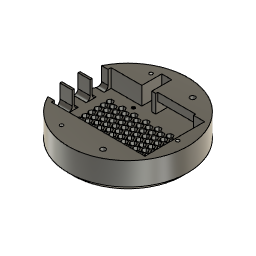
Lumo Base (Autodesk Fusion 360 design; units mm, degrees)
Autodesk Fusion 360 part; units mm, degrees
(part 1 of 2)
sketch "Pi Bounds" plane through (0, 0, 0) normal (0, 0, 1) x (1, 0, 0)
  circle A0 centre (0, 0) radius 60
  line L0 (-47, -30) -> (47, -30)
  line L1 (47, -30) -> (47, 30)
  line L2 (47, 30) -> (-47, 30)
  line L3 (-47, 30) -> (-47, -30)
  line L4 (-47, -30) -> (47, 30) construction
  line L5 (47, -30) -> (-47, 30) construction
  dimension "d1" = 60
  dimension "d2" = 94
  dimension "d3" = 120
  constraint coincident A0.centre origin
  constraint horizontal L0
  constraint perpendicular L0 L1
  constraint parallel L0 L2
  constraint parallel L1 L3
  constraint coincident L4 A0.centre
  constraint coincident L5 A0.centre
  measures "d1" distance of L0.end L1.end
  measures "d2" distance of L1.end L2.end
  measures "d3" diameter of A0
extrude "Extrude1" add sketch "Pi Bounds" along normal blind 28
extrude "Extrude2" add sketch "Pi Bounds" along normal blind 10 contours L0 L1 L2 L3
chamfer "Chamfer1" distance 5 angle 45 1 edges at (-55.9396, -21.6969, 0)
sketch "Screw Holes" plane through (0, 0, 10) normal (0, 0, 1) x (-1, 0, 0)
  line L0 (47, -30) -> (47, 30)
  line L1 (47, 30) -> (-47, 30)
  line L2 (-47, -30) -> (47, -30)
  line L3 (-47, -30) -> (-47, 30)
  point P0 (-39, 24.5)
  point P1 (-39, -24.5)
  point P2 (19, -24.5)
  point P3 (19, 24.5)
  dimension "d35" = 58
  dimension "d36" = 49
  dimension "d144" = 24.5
  dimension "d145" = 39
  dimension "d146" = 8
  constraint vertical P0 P1
  constraint horizontal P0 P3
  constraint vertical P2 P3
  constraint horizontal P1 P2
  measures "d35" distance of P0 P3
  measures "d36" distance of P0 P1
  measures "d144" vertical distance of origin P0
  measures "d145" horizontal distance of origin P0
  measures "d146" distance of P0 L3
hole "Hole3" at (-19, -24.5, 10) at (-19, 24.5, 10) at (39, 24.5, 10) at (39, -24.5, 10) direction (0, 0, -1) diameter 2.529 depth 6 tip angle 180
thread "Thread1" "ISO Metric profile 3.0 M3x0.5 6H" major diameter 3.086 minor diameter 2.529 pitch 0.5 angle 60 modelled right hand crest width 0.1368 on face at (-18.937, -25.7629, 8) crest through (-17.7355, -24.5, 9.875) on face at (-18.937, 23.2371, 8) crest through (-17.7355, 24.5, 9.875) on face at (38.3406, 23.421, 8) crest through (40.2645, 24.5, 9.875) on face at (38.2365, -25.508, 8) crest through (40.2645, -24.5, 9.875)
sketch "Access Holes (Side)" plane through (0, 30, 0) normal (0, -1, 0) x (1, 0, 0)
  line L0 (-47, 10) -> (47, 10)
  line L1 (47, 10) -> (47, 28)
  line L2 (47, 28) -> (-47, 28)
  line L3 (-47, 28) -> (-47, 10)
  line L4 (35.8, 20) -> (25.8, 20)
  line L5 (25.8, 20) -> (25.8, 10)
  line L6 (25.8, 10) -> (35.8, 10)
  line L7 (35.8, 10) -> (35.8, 20)
  line L8 (35.8, 20) -> (25.8, 10) construction
  line L9 (25.8, 20) -> (35.8, 10) construction
  line L10 (21, 10) -> (11, 10)
  line L11 (11, 10) -> (11, 20)
  line L12 (11, 20) -> (21, 20)
  line L13 (21, 20) -> (21, 10)
  line L14 (21, 10) -> (11, 20) construction
  line L15 (11, 10) -> (21, 20) construction
  line L16 (7.869, 20) -> (-2.131, 20)
  line L17 (-2.131, 20) -> (-2.131, 10)
  line L18 (-2.131, 10) -> (7.869, 10)
  line L19 (7.869, 10) -> (7.869, 20)
  line L20 (7.869, 20) -> (-2.131, 10) construction
  line L21 (-2.131, 20) -> (7.869, 10) construction
  line L22 (35.8, 10) -> (-2.131, 10)
  line L23 (-2.131, 10) -> (-2.131, 20)
  line L24 (-2.131, 20) -> (35.8, 20)
  line L25 (35.8, 20) -> (35.8, 10)
  point P0 (30.8, 15)
  point P1 (30.8, 15)
  point P2 (16, 15)
  point P3 (16, 15)
  point P4 (2.5, 15)
  point P5 (2.869, 15)
  dimension "d61" = 16.2
  dimension "d62" = 10
  dimension "d63" = 10
  dimension "d64" = 5
  dimension "d66" = 14.8
  dimension "d67" = 10
  dimension "d68" = 10
  dimension "d69" = 13.5
  dimension "d70" = 10
  dimension "d71" = 10
  constraint horizontal L4
  constraint perpendicular L4 L5
  constraint parallel L4 L6
  constraint parallel L5 L7
  constraint coincident L8 P1
  constraint coincident L9 P1
  constraint coincident P1 P0
  constraint horizontal P1 P3
  constraint horizontal L10
  constraint perpendicular L10 L11
  constraint parallel L10 L12
  constraint parallel L11 L13
  constraint coincident L14 P3
  constraint coincident L15 P3
  constraint coincident P3 P2
  constraint horizontal P3 P4
  constraint horizontal L16
  constraint perpendicular L16 L17
  constraint parallel L16 L18
  constraint parallel L17 L19
  constraint coincident L20 P5
  constraint coincident L21 P5
  constraint horizontal P3 P5
  constraint horizontal L22
  constraint vertical L23
  constraint horizontal L24
  constraint vertical L25
  measures "d61" distance of L1 P1
  measures "d62" distance of L5.end L6.end
  measures "d63" distance of L4.end L5.end
  measures "d64" distance of L0 P1
  measures "d66" distance of P1 P3
  measures "d67" distance of L11.end L12.end
  measures "d68" distance of L10.end L11.end
  measures "d69" distance of P3 P4
  measures "d70" distance of L17.end L18.end
  measures "d71" distance of L16.end L17.end
extrude "Extrude4" cut sketch "Access Holes (Side)" against normal through all contours L0 L16 L17 L18 L19 L22 L23 L24 | L0 L11 L19 L22 L24 | L0 L10 L11 L12 L13 L22 L24 | L0 L5 L13 L22 L24 | L0 L4 L5 L6 L7 L22 L24 L25
sketch "Connectors/Feet" plane through (0, 0, 0) normal (0, 0, -1) x (1, 0, 0)
  circle A0 centre (0, 0) radius 55
  circle A1 centre (0, 0) radius 50
  line L0 (40, -40) -> (-40, -40)
  line L1 (-40, -40) -> (-40, 40)
  line L2 (-40, 40) -> (40, 40)
  line L3 (40, 40) -> (40, -40)
  line L4 (40, -40) -> (-40, 40) construction
  line L5 (-40, -40) -> (40, 40) construction
  point P0 (50, 0)
  point P1 (-21.7945, 45)
  point P2 (-21.7945, -45)
  dimension "d138" = 100
  dimension "d141" = 45
  dimension "d142" = 80
  dimension "d143" = 80
  constraint coincident A0.centre A1.centre
  constraint coincident A1 P0
  constraint coincident A1 P1
  constraint vertical P1 P2
  constraint coincident A1 P2
  constraint horizontal L0
  constraint perpendicular L0 L1
  constraint parallel L0 L2
  constraint parallel L1 L3
  constraint coincident L4 A0.centre
  constraint coincident L5 A0.centre
  measures "d138" diameter of A1
  measures "d141" vertical distance of A0.centre P1
  measures "d142" distance of L1.end L2.end
  measures "d143" distance of L0.end L1.end
hole "Hole4" at (-21.7945, 45, 0) at (-21.7945, -45, 0) at (50, 0, 0) direction (0, 0, 1) diameter 3.332 end through all counterbore diameter 8 counterbore depth 2
thread "Thread2" "ISO Metric profile 4.0 M4x0.7 6H" major diameter 4.1095 minor diameter 3.332 pitch 0.7 angle 60 resizes the face on face at (-21.6286, -43.3423, 10.6667) on face at (50.1659, 1.6577, 10.6667) on face at (-21.6286, 46.6577, 10.6667)
sketch "Hexagon Air Holes" plane through (0, 0, 10) normal (0, 0, 1) x (-1, 0, 0)
  arc A0 (18.0419, 23.6748) -> (19.9581, 23.6748) centre (19, 24.5) ccw
  spline S0 degree 3 poles (18.0419, 23.6748) (17.9198, 23.7888) (17.8216, 23.926) (17.6793, 24.236) (17.6389, 24.407) (17.6243, 24.7618) (17.6529, 24.9423) (17.7788, 25.2891) (17.8774, 25.4512) (18.0844, 25.6792) (18.1756, 25.7577) (18.3768, 25.8929) (18.4864, 25.9486) (18.6015, 25.9906) knots 0 0 0 0 0.050111 0.050111 0.102261 0.102261 0.15645 0.15645 0.212677 0.212677 0.24852 0.24852 0.285143 0.285143 0.285143 0.285143
  arc A1 (-39.9581, 23.6748) -> (-38.0419, 23.6748) centre (-39, 24.5) ccw
  arc A2 (18.0419, -25.3252) -> (19.9581, -25.3252) centre (19, -24.5) ccw
  arc A3 (-39.9581, -25.3252) -> (-38.0419, -25.3252) centre (-39, -24.5) ccw
  line L0 (47, -30) -> (47, 30)
  line L1 (47, 30) -> (-47, 30)
  line L2 (-47, 30) -> (-47, -30)
  line L3 (-47, -30) -> (-35.8, -30)
  line L4 (33, -18.088) -> (34.5, -20.6861)
  line L5 (34.5, -20.6861) -> (37.5, -20.6861)
  line L6 (37.5, -20.6861) -> (39, -18.088)
  line L7 (39, -18.088) -> (37.5, -15.4899)
  line L8 (37.5, -15.4899) -> (34.5, -15.4899)
  line L9 (34.5, -15.4899) -> (33, -18.088)
  line L10 (34.5, -14.4901) -> (37.5, -14.4901)
  line L11 (37.5, -14.4901) -> (39, -11.892)
  line L12 (39, -11.892) -> (37.5, -9.2939)
  line L13 (37.5, -9.2939) -> (34.5, -9.2939)
  line L14 (34.5, -9.2939) -> (33, -11.892)
  line L15 (33, -11.892) -> (34.5, -14.4901)
  line L16 (34.5, -8.2941) -> (37.5, -8.2941)
  line L17 (37.5, -8.2941) -> (39, -5.696)
  line L18 (39, -5.696) -> (37.5, -3.0979)
  line L19 (37.5, -3.0979) -> (34.5, -3.0979)
  line L20 (34.5, -3.0979) -> (33, -5.696)
  line L21 (33, -5.696) -> (34.5, -8.2941)
  line L22 (34.5, -2.0981) -> (37.5, -2.0981)
  line L23 (37.5, -2.0981) -> (39, 0.5)
  line L24 (39, 0.5) -> (37.5, 3.0981)
  line L25 (37.5, 3.0981) -> (34.5, 3.0981)
  line L26 (34.5, 3.0981) -> (33, 0.5)
  line L27 (33, 0.5) -> (34.5, -2.0981)
  line L28 (34.5, 4.0979) -> (37.5, 4.0979)
  line L29 (37.5, 4.0979) -> (39, 6.696)
  line L30 (39, 6.696) -> (37.5, 9.2941)
  line L31 (37.5, 9.2941) -> (34.5, 9.2941)
  line L32 (34.5, 9.2941) -> (33, 6.696)
  line L33 (33, 6.696) -> (34.5, 4.0979)
  line L34 (34.5, 10.2939) -> (37.5, 10.2939)
  line L35 (37.5, 10.2939) -> (39, 12.892)
  line L36 (39, 12.892) -> (37.5, 15.4901)
  line L37 (37.5, 15.4901) -> (34.5, 15.4901)
  line L38 (34.5, 15.4901) -> (33, 12.892)
  line L39 (33, 12.892) -> (34.5, 10.2939)
  line L40 (34.5, 16.4899) -> (37.5, 16.4899)
  line L41 (37.5, 16.4899) -> (39, 19.088)
  line L42 (39, 19.088) -> (37.5, 21.6861)
  line L43 (37.5, 21.6861) -> (34.5, 21.6861)
  line L44 (34.5, 21.6861) -> (33, 19.088)
  line L45 (33, 19.088) -> (34.5, 16.4899)
  line L46 (21, -18.088) -> (22.5, -20.6861)
  line L47 (22.5, -20.6861) -> (25.5, -20.6861)
  line L48 (25.5, -20.6861) -> (27, -18.088)
  line L49 (27, -18.088) -> (25.5, -15.4899)
  line L50 (22.5, -15.4899) -> (21, -18.088)
  line L51 (25.5, -15.4899) -> (22.5, -15.4899)
  line L52 (25.5, -9.2939) -> (22.5, -9.2939)
  line L53 (22.5, -9.2939) -> (21, -11.892)
  line L54 (21, -11.892) -> (22.5, -14.4901)
  line L55 (22.5, -14.4901) -> (25.5, -14.4901)
  line L56 (27, -11.892) -> (25.5, -9.2939)
  line L57 (25.5, -14.4901) -> (27, -11.892)
  line L58 (25.5, -3.0979) -> (22.5, -3.0979)
  line L59 (22.5, -3.0979) -> (21, -5.696)
  line L60 (21, -5.696) -> (22.5, -8.2941)
  line L61 (22.5, -8.2941) -> (25.5, -8.2941)
  line L62 (27, -5.696) -> (25.5, -3.0979)
  line L63 (25.5, -8.2941) -> (27, -5.696)
  line L64 (25.5, 3.0981) -> (22.5, 3.0981)
  line L65 (22.5, 3.0981) -> (21, 0.5)
  line L66 (21, 0.5) -> (22.5, -2.0981)
  line L67 (22.5, -2.0981) -> (25.5, -2.0981)
  line L68 (27, 0.5) -> (25.5, 3.0981)
  line L69 (25.5, -2.0981) -> (27, 0.5)
  line L70 (27, 6.696) -> (25.5, 9.2941)
  line L71 (25.5, 9.2941) -> (22.5, 9.2941)
  line L72 (22.5, 9.2941) -> (21, 6.696)
  line L73 (21, 6.696) -> (22.5, 4.0979)
  line L74 (25.5, 4.0979) -> (27, 6.696)
  line L75 (22.5, 4.0979) -> (25.5, 4.0979)
  line L76 (27, 12.892) -> (25.5, 15.4901)
  line L77 (25.5, 15.4901) -> (22.5, 15.4901)
  line L78 (22.5, 15.4901) -> (21, 12.892)
  line L79 (21, 12.892) -> (22.5, 10.2939)
  line L80 (25.5, 10.2939) -> (27, 12.892)
  line L81 (22.5, 10.2939) -> (25.5, 10.2939)
  line L82 (27, 19.088) -> (25.5, 21.6861)
  line L83 (25.5, 21.6861) -> (22.5, 21.6861)
  line L84 (22.5, 21.6861) -> (21, 19.088)
  line L85 (21, 19.088) -> (22.5, 16.4899)
  line L86 (25.5, 16.4899) -> (27, 19.088)
  line L87 (22.5, 16.4899) -> (25.5, 16.4899)
  line L88 (9, -18.088) -> (10.5, -20.6861)
  line L89 (10.5, -20.6861) -> (13.5, -20.6861)
  line L90 (13.5, -20.6861) -> (15, -18.088)
  line L91 (15, -18.088) -> (13.5, -15.4899)
  line L92 (10.5, -15.4899) -> (9, -18.088)
  line L93 (13.5, -15.4899) -> (10.5, -15.4899)
  line L94 (13.5, -9.2939) -> (10.5, -9.2939)
  line L95 (10.5, -9.2939) -> (9, -11.892)
  line L96 (9, -11.892) -> (10.5, -14.4901)
  line L97 (10.5, -14.4901) -> (13.5, -14.4901)
  line L98 (15, -11.892) -> (13.5, -9.2939)
  line L99 (13.5, -14.4901) -> (15, -11.892)
  line L100 (13.5, -3.0979) -> (10.5, -3.0979)
  line L101 (10.5, -3.0979) -> (9, -5.696)
  line L102 (9, -5.696) -> (10.5, -8.2941)
  line L103 (10.5, -8.2941) -> (13.5, -8.2941)
  line L104 (15, -5.696) -> (13.5, -3.0979)
  line L105 (13.5, -8.2941) -> (15, -5.696)
  line L106 (13.5, 3.0981) -> (10.5, 3.0981)
  line L107 (10.5, 3.0981) -> (9, 0.5)
  line L108 (9, 0.5) -> (10.5, -2.0981)
  line L109 (10.5, -2.0981) -> (13.5, -2.0981)
  line L110 (15, 0.5) -> (13.5, 3.0981)
  line L111 (13.5, -2.0981) -> (15, 0.5)
  line L112 (15, 6.696) -> (13.5, 9.2941)
  line L113 (13.5, 9.2941) -> (10.5, 9.2941)
  line L114 (10.5, 9.2941) -> (9, 6.696)
  line L115 (9, 6.696) -> (10.5, 4.0979)
  line L116 (13.5, 4.0979) -> (15, 6.696)
  line L117 (10.5, 4.0979) -> (13.5, 4.0979)
  line L118 (15, 12.892) -> (13.5, 15.4901)
  line L119 (13.5, 15.4901) -> (10.5, 15.4901)
  line L120 (10.5, 15.4901) -> (9, 12.892)
  line L121 (9, 12.892) -> (10.5, 10.2939)
  line L122 (13.5, 10.2939) -> (15, 12.892)
  line L123 (10.5, 10.2939) -> (13.5, 10.2939)
  line L124 (15, 19.088) -> (13.5, 21.6861)
  line L125 (13.5, 21.6861) -> (10.5, 21.6861)
  line L126 (10.5, 21.6861) -> (9, 19.088)
  line L127 (9, 19.088) -> (10.5, 16.4899)
  line L128 (13.5, 16.4899) -> (15, 19.088)
  line L129 (10.5, 16.4899) -> (13.5, 16.4899)
  line L130 (-3, -18.088) -> (-1.5, -20.6861)
  line L131 (-1.5, -20.6861) -> (1.5, -20.6861)
  line L132 (1.5, -20.6861) -> (3, -18.088)
  line L133 (3, -18.088) -> (1.5, -15.4899)
  line L134 (-1.5, -15.4899) -> (-3, -18.088)
  line L135 (1.5, -15.4899) -> (-1.5, -15.4899)
  line L136 (1.5, -9.2939) -> (-1.5, -9.2939)
  line L137 (-1.5, -9.2939) -> (-3, -11.892)
  line L138 (-3, -11.892) -> (-1.5, -14.4901)
  line L139 (-1.5, -14.4901) -> (1.5, -14.4901)
  line L140 (3, -11.892) -> (1.5, -9.2939)
  line L141 (1.5, -14.4901) -> (3, -11.892)
  line L142 (1.5, -3.0979) -> (-1.5, -3.0979)
  line L143 (-1.5, -3.0979) -> (-3, -5.696)
  line L144 (-3, -5.696) -> (-1.5, -8.2941)
  line L145 (-1.5, -8.2941) -> (1.5, -8.2941)
  line L146 (3, -5.696) -> (1.5, -3.0979)
  line L147 (1.5, -8.2941) -> (3, -5.696)
  line L148 (1.5, 3.0981) -> (-1.5, 3.0981)
  line L149 (-1.5, 3.0981) -> (-3, 0.5)
  line L150 (-3, 0.5) -> (-1.5, -2.0981)
  line L151 (-1.5, -2.0981) -> (1.5, -2.0981)
  line L152 (3, 0.5) -> (1.5, 3.0981)
  line L153 (1.5, -2.0981) -> (3, 0.5)
  line L154 (3, 6.696) -> (1.5, 9.2941)
  line L155 (1.5, 9.2941) -> (-1.5, 9.2941)
  line L156 (-1.5, 9.2941) -> (-3, 6.696)
  line L157 (-3, 6.696) -> (-1.5, 4.0979)
  line L158 (1.5, 4.0979) -> (3, 6.696)
  line L159 (-1.5, 4.0979) -> (1.5, 4.0979)
  line L160 (3, 12.892) -> (1.5, 15.4901)
  line L161 (1.5, 15.4901) -> (-1.5, 15.4901)
  line L162 (-1.5, 15.4901) -> (-3, 12.892)
  line L163 (-3, 12.892) -> (-1.5, 10.2939)
  line L164 (1.5, 10.2939) -> (3, 12.892)
  line L165 (-1.5, 10.2939) -> (1.5, 10.2939)
  line L166 (3, 19.088) -> (1.5, 21.6861)
  line L167 (1.5, 21.6861) -> (-1.5, 21.6861)
  line L168 (-1.5, 21.6861) -> (-3, 19.088)
  line L169 (-3, 19.088) -> (-1.5, 16.4899)
  line L170 (1.5, 16.4899) -> (3, 19.088)
  line L171 (-1.5, 16.4899) -> (1.5, 16.4899)
  line L172 (-15, -18.088) -> (-13.5, -20.6861)
  line L173 (-13.5, -20.6861) -> (-10.5, -20.6861)
  line L174 (-10.5, -20.6861) -> (-9, -18.088)
  line L175 (-9, -18.088) -> (-10.5, -15.4899)
  line L176 (-13.5, -15.4899) -> (-15, -18.088)
  line L177 (-10.5, -15.4899) -> (-13.5, -15.4899)
  line L178 (-10.5, -9.2939) -> (-13.5, -9.2939)
  line L179 (-13.5, -9.2939) -> (-15, -11.892)
  line L180 (-15, -11.892) -> (-13.5, -14.4901)
  line L181 (-13.5, -14.4901) -> (-10.5, -14.4901)
  line L182 (-9, -11.892) -> (-10.5, -9.2939)
  line L183 (-10.5, -14.4901) -> (-9, -11.892)
  line L184 (-10.5, -3.0979) -> (-13.5, -3.0979)
  line L185 (-13.5, -3.0979) -> (-15, -5.696)
  line L186 (-15, -5.696) -> (-13.5, -8.2941)
  line L187 (-13.5, -8.2941) -> (-10.5, -8.2941)
  line L188 (-9, -5.696) -> (-10.5, -3.0979)
  line L189 (-10.5, -8.2941) -> (-9, -5.696)
  line L190 (-10.5, 3.0981) -> (-13.5, 3.0981)
  line L191 (-13.5, 3.0981) -> (-15, 0.5)
  line L192 (-15, 0.5) -> (-13.5, -2.0981)
  line L193 (-13.5, -2.0981) -> (-10.5, -2.0981)
  line L194 (-9, 0.5) -> (-10.5, 3.0981)
  line L195 (-10.5, -2.0981) -> (-9, 0.5)
  line L196 (-9, 6.696) -> (-10.5, 9.2941)
  line L197 (-10.5, 9.2941) -> (-13.5, 9.2941)
  line L198 (-13.5, 9.2941) -> (-15, 6.696)
  line L199 (-15, 6.696) -> (-13.5, 4.0979)
  line L200 (-10.5, 4.0979) -> (-9, 6.696)
  line L201 (-13.5, 4.0979) -> (-10.5, 4.0979)
  line L202 (-9, 12.892) -> (-10.5, 15.4901)
  line L203 (-10.5, 15.4901) -> (-13.5, 15.4901)
  line L204 (-13.5, 15.4901) -> (-15, 12.892)
  line L205 (-15, 12.892) -> (-13.5, 10.2939)
  line L206 (-10.5, 10.2939) -> (-9, 12.892)
  line L207 (-13.5, 10.2939) -> (-10.5, 10.2939)
  line L208 (-9, 19.088) -> (-10.5, 21.6861)
  line L209 (-10.5, 21.6861) -> (-13.5, 21.6861)
  line L210 (-13.5, 21.6861) -> (-15, 19.088)
  line L211 (-15, 19.088) -> (-13.5, 16.4899)
  line L212 (-10.5, 16.4899) -> (-9, 19.088)
  line L213 (-13.5, 16.4899) -> (-10.5, 16.4899)
  line L214 (-27, -18.088) -> (-25.5, -20.6861)
  line L215 (-25.5, -20.6861) -> (-22.5, -20.6861)
  line L216 (-22.5, -20.6861) -> (-21, -18.088)
  line L217 (-21, -18.088) -> (-22.5, -15.4899)
  line L218 (-25.5, -15.4899) -> (-27, -18.088)
  line L219 (-22.5, -15.4899) -> (-25.5, -15.4899)
  line L220 (-22.5, -9.2939) -> (-25.5, -9.2939)
  line L221 (-25.5, -9.2939) -> (-27, -11.892)
  line L222 (-27, -11.892) -> (-25.5, -14.4901)
  line L223 (-25.5, -14.4901) -> (-22.5, -14.4901)
  line L224 (-21, -11.892) -> (-22.5, -9.2939)
  line L225 (-22.5, -14.4901) -> (-21, -11.892)
  line L226 (-22.5, -3.0979) -> (-25.5, -3.0979)
  line L227 (-25.5, -3.0979) -> (-27, -5.696)
  line L228 (-27, -5.696) -> (-25.5, -8.2941)
  line L229 (-25.5, -8.2941) -> (-22.5, -8.2941)
  line L230 (-21, -5.696) -> (-22.5, -3.0979)
  line L231 (-22.5, -8.2941) -> (-21, -5.696)
  line L232 (-22.5, 3.0981) -> (-25.5, 3.0981)
  line L233 (-25.5, 3.0981) -> (-27, 0.5)
  line L234 (-27, 0.5) -> (-25.5, -2.0981)
  line L235 (-25.5, -2.0981) -> (-22.5, -2.0981)
  line L236 (-21, 0.5) -> (-22.5, 3.0981)
  line L237 (-22.5, -2.0981) -> (-21, 0.5)
  line L238 (-21, 6.696) -> (-22.5, 9.2941)
  line L239 (-22.5, 9.2941) -> (-25.5, 9.2941)
  line L240 (-25.5, 9.2941) -> (-27, 6.696)
  line L241 (-27, 6.696) -> (-25.5, 4.0979)
  line L242 (-22.5, 4.0979) -> (-21, 6.696)
  line L243 (-25.5, 4.0979) -> (-22.5, 4.0979)
  line L244 (-21, 12.892) -> (-22.5, 15.4901)
  line L245 (-22.5, 15.4901) -> (-25.5, 15.4901)
  line L246 (-25.5, 15.4901) -> (-27, 12.892)
  line L247 (-27, 12.892) -> (-25.5, 10.2939)
  line L248 (-22.5, 10.2939) -> (-21, 12.892)
  line L249 (-25.5, 10.2939) -> (-22.5, 10.2939)
  line L250 (-21, 19.088) -> (-22.5, 21.6861)
  line L251 (-22.5, 21.6861) -> (-25.5, 21.6861)
  line L252 (-25.5, 21.6861) -> (-27, 19.088)
  line L253 (-27, 19.088) -> (-25.5, 16.4899)
  line L254 (-22.5, 16.4899) -> (-21, 19.088)
  line L255 (-25.5, 16.4899) -> (-22.5, 16.4899)
  line L256 (31.5, -17.5881) -> (33, -14.99)
  line L257 (33, -14.99) -> (31.5, -12.3919)
  line L258 (31.5, -12.3919) -> (28.5, -12.3919)
  line L259 (28.5, -12.3919) -> (27, -14.99)
  line L260 (27, -14.99) -> (28.5, -17.5881)
  line L261 (28.5, -17.5881) -> (31.5, -17.5881)
  line L262 (-47, -30) -> (47, -30)
  line L263 (30, -14.99) -> (36, -18.088)
  line L264 (25.5, -20.6861) -> (22.5, -15.4899)
  line L265 (30, -14.99) -> (24, -18.088)
  line L266 (37.5, -14.4901) -> (34.5, -9.2939)
  line L267 (36, -11.892) -> (30, -14.99)
  line L268 (15, -14.99) -> (16.5, -17.5881)
  line L269 (16.5, -17.5881) -> (19.5, -17.5881)
  line L270 (19.5, -17.5881) -> (21, -14.99)
  line L271 (21, -14.99) -> (19.5, -12.3919)
  line L272 (16.5, -12.3919) -> (15, -14.99)
  line L273 (19.5, -12.3919) -> (16.5, -12.3919)
  line L274 (3, -14.99) -> (4.5, -17.5881)
  line L275 (4.5, -17.5881) -> (7.5, -17.5881)
  line L276 (7.5, -17.5881) -> (9, -14.99)
  line L277 (9, -14.99) -> (7.5, -12.3919)
  line L278 (4.5, -12.3919) -> (3, -14.99)
  line L279 (7.5, -12.3919) -> (4.5, -12.3919)
  line L280 (-9, -14.99) -> (-7.5, -17.5881)
  line L281 (-7.5, -17.5881) -> (-4.5, -17.5881)
  line L282 (-4.5, -17.5881) -> (-3, -14.99)
  line L283 (-3, -14.99) -> (-4.5, -12.3919)
  line L284 (-7.5, -12.3919) -> (-9, -14.99)
  line L285 (-4.5, -12.3919) -> (-7.5, -12.3919)
  line L286 (-21, -14.99) -> (-19.5, -17.5881)
  line L287 (-19.5, -17.5881) -> (-16.5, -17.5881)
  line L288 (-16.5, -17.5881) -> (-15, -14.99)
  line L289 (-15, -14.99) -> (-16.5, -12.3919)
  line L290 (-19.5, -12.3919) -> (-21, -14.99)
  line L291 (-16.5, -12.3919) -> (-19.5, -12.3919)
  line L292 (-33, -14.99) -> (-31.5, -17.5881)
  line L293 (-31.5, -17.5881) -> (-28.5, -17.5881)
  line L294 (-28.5, -17.5881) -> (-27, -14.99)
  line L295 (-27, -14.99) -> (-28.5, -12.3919)
  line L296 (-31.5, -12.3919) -> (-33, -14.99)
  line L297 (-28.5, -12.3919) -> (-31.5, -12.3919)
  line L298 (27, -8.821) -> (28.5, -11.4191)
  line L299 (28.5, -11.4191) -> (31.5, -11.4191)
  line L300 (31.5, -11.4191) -> (33, -8.821)
  line L301 (33, -8.821) -> (31.5, -6.2229)
  line L302 (28.5, -6.2229) -> (27, -8.821)
  line L303 (31.5, -6.2229) -> (28.5, -6.2229)
  line L304 (15, -8.821) -> (16.5, -11.4191)
  line L305 (16.5, -11.4191) -> (19.5, -11.4191)
  line L306 (19.5, -11.4191) -> (21, -8.821)
  line L307 (21, -8.821) -> (19.5, -6.2229)
  line L308 (16.5, -6.2229) -> (15, -8.821)
  line L309 (19.5, -6.2229) -> (16.5, -6.2229)
  line L310 (3, -8.821) -> (4.5, -11.4191)
  line L311 (4.5, -11.4191) -> (7.5, -11.4191)
  line L312 (7.5, -11.4191) -> (9, -8.821)
  line L313 (9, -8.821) -> (7.5, -6.2229)
  line L314 (4.5, -6.2229) -> (3, -8.821)
  line L315 (7.5, -6.2229) -> (4.5, -6.2229)
  line L316 (-9, -8.821) -> (-7.5, -11.4191)
  line L317 (-7.5, -11.4191) -> (-4.5, -11.4191)
  line L318 (-4.5, -11.4191) -> (-3, -8.821)
  line L319 (-3, -8.821) -> (-4.5, -6.2229)
  line L320 (-7.5, -6.2229) -> (-9, -8.821)
  line L321 (-4.5, -6.2229) -> (-7.5, -6.2229)
  line L322 (-21, -8.821) -> (-19.5, -11.4191)
  line L323 (-19.5, -11.4191) -> (-16.5, -11.4191)
  line L324 (-16.5, -11.4191) -> (-15, -8.821)
  line L325 (-15, -8.821) -> (-16.5, -6.2229)
  line L326 (-19.5, -6.2229) -> (-21, -8.821)
  line L327 (-16.5, -6.2229) -> (-19.5, -6.2229)
  line L328 (-33, -8.821) -> (-31.5, -11.4191)
  line L329 (-31.5, -11.4191) -> (-28.5, -11.4191)
  line L330 (-28.5, -11.4191) -> (-27, -8.821)
  line L331 (-27, -8.821) -> (-28.5, -6.2229)
  line L332 (-31.5, -6.2229) -> (-33, -8.821)
  line L333 (-28.5, -6.2229) -> (-31.5, -6.2229)
  line L334 (27, -2.652) -> (28.5, -5.2501)
  line L335 (28.5, -5.2501) -> (31.5, -5.2501)
  line L336 (31.5, -5.2501) -> (33, -2.652)
  line L337 (33, -2.652) -> (31.5, -0.0539)
  line L338 (28.5, -0.0539) -> (27, -2.652)
  line L339 (31.5, -0.0539) -> (28.5, -0.0539)
  line L340 (15, -2.652) -> (16.5, -5.2501)
  line L341 (16.5, -5.2501) -> (19.5, -5.2501)
  line L342 (19.5, -5.2501) -> (21, -2.652)
  line L343 (21, -2.652) -> (19.5, -0.0539)
  line L344 (16.5, -0.0539) -> (15, -2.652)
  line L345 (19.5, -0.0539) -> (16.5, -0.0539)
  line L346 (3, -2.652) -> (4.5, -5.2501)
  line L347 (4.5, -5.2501) -> (7.5, -5.2501)
  line L348 (7.5, -5.2501) -> (9, -2.652)
  line L349 (9, -2.652) -> (7.5, -0.0539)
  line L350 (4.5, -0.0539) -> (3, -2.652)
  line L351 (7.5, -0.0539) -> (4.5, -0.0539)
  line L352 (-9, -2.652) -> (-7.5, -5.2501)
  line L353 (-7.5, -5.2501) -> (-4.5, -5.2501)
  line L354 (-4.5, -5.2501) -> (-3, -2.652)
  line L355 (-3, -2.652) -> (-4.5, -0.0539)
  line L356 (-7.5, -0.0539) -> (-9, -2.652)
  line L357 (-4.5, -0.0539) -> (-7.5, -0.0539)
  line L358 (-21, -2.652) -> (-19.5, -5.2501)
  line L359 (-19.5, -5.2501) -> (-16.5, -5.2501)
  line L360 (-16.5, -5.2501) -> (-15, -2.652)
  line L361 (-15, -2.652) -> (-16.5, -0.0539)
  line L362 (-19.5, -0.0539) -> (-21, -2.652)
  line L363 (-16.5, -0.0539) -> (-19.5, -0.0539)
  line L364 (-33, -2.652) -> (-31.5, -5.2501)
  line L365 (-31.5, -5.2501) -> (-28.5, -5.2501)
  line L366 (-28.5, -5.2501) -> (-27, -2.652)
  line L367 (-27, -2.652) -> (-28.5, -0.0539)
  line L368 (-31.5, -0.0539) -> (-33, -2.652)
  line L369 (-28.5, -0.0539) -> (-31.5, -0.0539)
  line L370 (27, 3.517) -> (28.5, 0.9189)
  line L371 (28.5, 0.9189) -> (31.5, 0.9189)
  line L372 (31.5, 0.9189) -> (33, 3.517)
  line L373 (33, 3.517) -> (31.5, 6.1151)
  line L374 (28.5, 6.1151) -> (27, 3.517)
  line L375 (31.5, 6.1151) -> (28.5, 6.1151)
  line L376 (15, 3.517) -> (16.5, 0.9189)
  line L377 (16.5, 0.9189) -> (19.5, 0.9189)
  line L378 (19.5, 0.9189) -> (21, 3.517)
  line L379 (21, 3.517) -> (19.5, 6.1151)
  line L380 (16.5, 6.1151) -> (15, 3.517)
  line L381 (19.5, 6.1151) -> (16.5, 6.1151)
  line L382 (3, 3.517) -> (4.5, 0.9189)
  line L383 (4.5, 0.9189) -> (7.5, 0.9189)
  line L384 (7.5, 0.9189) -> (9, 3.517)
  line L385 (9, 3.517) -> (7.5, 6.1151)
  line L386 (4.5, 6.1151) -> (3, 3.517)
  line L387 (7.5, 6.1151) -> (4.5, 6.1151)
  line L388 (-9, 3.517) -> (-7.5, 0.9189)
  line L389 (-7.5, 0.9189) -> (-4.5, 0.9189)
  line L390 (-4.5, 0.9189) -> (-3, 3.517)
  line L391 (-3, 3.517) -> (-4.5, 6.1151)
  line L392 (-7.5, 6.1151) -> (-9, 3.517)
  line L393 (-4.5, 6.1151) -> (-7.5, 6.1151)
  line L394 (-21, 3.517) -> (-19.5, 0.9189)
  line L395 (-19.5, 0.9189) -> (-16.5, 0.9189)
  line L396 (-16.5, 0.9189) -> (-15, 3.517)
  line L397 (-15, 3.517) -> (-16.5, 6.1151)
  line L398 (-19.5, 6.1151) -> (-21, 3.517)
  line L399 (-16.5, 6.1151) -> (-19.5, 6.1151)
  line L400 (-33, 3.517) -> (-31.5, 0.9189)
  line L401 (-31.5, 0.9189) -> (-28.5, 0.9189)
  line L402 (-28.5, 0.9189) -> (-27, 3.517)
  line L403 (-27, 3.517) -> (-28.5, 6.1151)
  line L404 (-31.5, 6.1151) -> (-33, 3.517)
  line L405 (-28.5, 6.1151) -> (-31.5, 6.1151)
  line L406 (27, 9.686) -> (28.5, 7.0879)
  line L407 (28.5, 7.0879) -> (31.5, 7.0879)
  line L408 (31.5, 7.0879) -> (33, 9.686)
  line L409 (33, 9.686) -> (31.5, 12.2841)
  line L410 (28.5, 12.2841) -> (27, 9.686)
  line L411 (31.5, 12.2841) -> (28.5, 12.2841)
  line L412 (15, 9.686) -> (16.5, 7.0879)
  line L413 (16.5, 7.0879) -> (19.5, 7.0879)
  line L414 (19.5, 7.0879) -> (21, 9.686)
  line L415 (21, 9.686) -> (19.5, 12.2841)
  line L416 (16.5, 12.2841) -> (15, 9.686)
  line L417 (19.5, 12.2841) -> (16.5, 12.2841)
  line L418 (3, 9.686) -> (4.5, 7.0879)
  line L419 (4.5, 7.0879) -> (7.5, 7.0879)
  line L420 (7.5, 7.0879) -> (9, 9.686)
  line L421 (9, 9.686) -> (7.5, 12.2841)
  line L422 (4.5, 12.2841) -> (3, 9.686)
  line L423 (7.5, 12.2841) -> (4.5, 12.2841)
  line L424 (-9, 9.686) -> (-7.5, 7.0879)
  line L425 (-7.5, 7.0879) -> (-4.5, 7.0879)
  line L426 (-4.5, 7.0879) -> (-3, 9.686)
  line L427 (-3, 9.686) -> (-4.5, 12.2841)
  line L428 (-7.5, 12.2841) -> (-9, 9.686)
  line L429 (-4.5, 12.2841) -> (-7.5, 12.2841)
  line L430 (-21, 9.686) -> (-19.5, 7.0879)
  line L431 (-19.5, 7.0879) -> (-16.5, 7.0879)
  line L432 (-16.5, 7.0879) -> (-15, 9.686)
  line L433 (-15, 9.686) -> (-16.5, 12.2841)
  line L434 (-19.5, 12.2841) -> (-21, 9.686)
  line L435 (-16.5, 12.2841) -> (-19.5, 12.2841)
  line L436 (-33, 9.686) -> (-31.5, 7.0879)
  line L437 (-31.5, 7.0879) -> (-28.5, 7.0879)
  line L438 (-28.5, 7.0879) -> (-27, 9.686)
  line L439 (-27, 9.686) -> (-28.5, 12.2841)
  line L440 (-31.5, 12.2841) -> (-33, 9.686)
  line L441 (-28.5, 12.2841) -> (-31.5, 12.2841)
  line L442 (27, 15.855) -> (28.5, 13.2569)
  line L443 (28.5, 13.2569) -> (31.5, 13.2569)
  line L444 (31.5, 13.2569) -> (33, 15.855)
  line L445 (33, 15.855) -> (31.5, 18.4531)
  line L446 (28.5, 18.4531) -> (27, 15.855)
  line L447 (31.5, 18.4531) -> (28.5, 18.4531)
  line L448 (15, 15.855) -> (16.5, 13.2569)
  line L449 (16.5, 13.2569) -> (19.5, 13.2569)
  line L450 (19.5, 13.2569) -> (21, 15.855)
  line L451 (21, 15.855) -> (19.5, 18.4531)
  line L452 (16.5, 18.4531) -> (15, 15.855)
  line L453 (19.5, 18.4531) -> (16.5, 18.4531)
  line L454 (3, 15.855) -> (4.5, 13.2569)
  line L455 (4.5, 13.2569) -> (7.5, 13.2569)
  line L456 (7.5, 13.2569) -> (9, 15.855)
  line L457 (9, 15.855) -> (7.5, 18.4531)
  line L458 (4.5, 18.4531) -> (3, 15.855)
  line L459 (7.5, 18.4531) -> (4.5, 18.4531)
  line L460 (-9, 15.855) -> (-7.5, 13.2569)
  line L461 (-7.5, 13.2569) -> (-4.5, 13.2569)
  line L462 (-4.5, 13.2569) -> (-3, 15.855)
  line L463 (-3, 15.855) -> (-4.5, 18.4531)
  line L464 (-7.5, 18.4531) -> (-9, 15.855)
  line L465 (-4.5, 18.4531) -> (-7.5, 18.4531)
  line L466 (-21, 15.855) -> (-19.5, 13.2569)
  line L467 (-19.5, 13.2569) -> (-16.5, 13.2569)
  line L468 (-16.5, 13.2569) -> (-15, 15.855)
  line L469 (-15, 15.855) -> (-16.5, 18.4531)
  line L470 (-19.5, 18.4531) -> (-21, 15.855)
  line L471 (-16.5, 18.4531) -> (-19.5, 18.4531)
  line L472 (-33, 15.855) -> (-31.5, 13.2569)
  line L473 (-31.5, 13.2569) -> (-28.5, 13.2569)
  line L474 (-28.5, 13.2569) -> (-27, 15.855)
  line L475 (-27, 15.855) -> (-28.5, 18.4531)
  line L476 (-31.5, 18.4531) -> (-33, 15.855)
  line L477 (-28.5, 18.4531) -> (-31.5, 18.4531)
  line L478 (47, -30) -> (47, 30)
  arc A4 (19.3985, 25.9906) -> (18.6015, 25.9906) centre (19, 24.5) ccw
  spline S1 degree 3 poles (-38.6015, 25.9906) (-38.4166, 25.9231) (-38.2465, 25.8207) (-37.9611, 25.5601) (-37.8468, 25.4065) (-37.6876, 25.0696) (-37.6419, 24.8908) (-37.6233, 24.5326) (-37.648, 24.3568) (-37.741, 24.0918) (-37.7875, 23.9972) (-37.901, 23.8235) (-37.967, 23.7447) (-38.0419, 23.6748) knots 0 0 0 0 0.059039 0.059039 0.116033 0.116033 0.170983 0.170983 0.223888 0.223888 0.255505 0.255505 0.286347 0.286347 0.286347 0.286347
  spline S2 degree 3 poles (-39.9581, 23.6748) (-40.0802, 23.7888) (-40.1784, 23.926) (-40.3207, 24.236) (-40.3611, 24.407) (-40.3757, 24.7618) (-40.3471, 24.9423) (-40.2212, 25.2891) (-40.1226, 25.4512) (-39.9156, 25.6792) (-39.8244, 25.7577) (-39.6232, 25.8929) (-39.5136, 25.9486) (-39.3985, 25.9906) knots 0 0 0 0 0.050111 0.050111 0.102261 0.102261 0.15645 0.15645 0.212677 0.212677 0.24852 0.24852 0.285143 0.285143 0.285143 0.285143
  spline S3 degree 3 poles (-38.6015, -23.0094) (-38.4166, -23.0769) (-38.2465, -23.1793) (-37.9611, -23.4399) (-37.8468, -23.5935) (-37.6876, -23.9304) (-37.6419, -24.1092) (-37.6233, -24.4674) (-37.648, -24.6432) (-37.741, -24.9082) (-37.7875, -25.0028) (-37.901, -25.1765) (-37.967, -25.2553) (-38.0419, -25.3252) knots 0 0 0 0 0.059039 0.059039 0.116033 0.116033 0.170983 0.170983 0.223888 0.223888 0.255505 0.255505 0.286347 0.286347 0.286347 0.286347
  spline S4 degree 3 poles (-39.9581, -25.3252) (-40.0802, -25.2112) (-40.1784, -25.074) (-40.3207, -24.764) (-40.3611, -24.593) (-40.3757, -24.2382) (-40.3471, -24.0577) (-40.2212, -23.7109) (-40.1226, -23.5488) (-39.9156, -23.3208) (-39.8244, -23.2423) (-39.6232, -23.1071) (-39.5136, -23.0514) (-39.3985, -23.0094) knots 0 0 0 0 0.050111 0.050111 0.102261 0.102261 0.15645 0.15645 0.212677 0.212677 0.24852 0.24852 0.285143 0.285143 0.285143 0.285143
  spline S5 degree 3 poles (19.3985, -23.0094) (19.5834, -23.0769) (19.7535, -23.1793) (20.0389, -23.4399) (20.1532, -23.5935) (20.3124, -23.9304) (20.3581, -24.1092) (20.3767, -24.4674) (20.352, -24.6432) (20.259, -24.9082) (20.2125, -25.0028) (20.099, -25.1765) (20.033, -25.2553) (19.9581, -25.3252) knots 0 0 0 0 0.059039 0.059039 0.116033 0.116033 0.170983 0.170983 0.223888 0.223888 0.255505 0.255505 0.286347 0.286347 0.286347 0.286347
  spline S6 degree 3 poles (18.0419, -25.3252) (17.9198, -25.2112) (17.8216, -25.074) (17.6793, -24.764) (17.6389, -24.593) (17.6243, -24.2382) (17.6529, -24.0577) (17.7788, -23.7109) (17.8774, -23.5488) (18.0844, -23.3208) (18.1756, -23.2423) (18.3768, -23.1071) (18.4864, -23.0514) (18.6015, -23.0094) knots 0 0 0 0 0.050111 0.050111 0.102261 0.102261 0.15645 0.15645 0.212677 0.212677 0.24852 0.24852 0.285143 0.285143 0.285143 0.285143
  line L479 (-35.8, -30) -> (-35.8, -48.1494)
  arc A5 (-35.8, -48.1494) -> (2.131, -59.9621) centre (0, 0) ccw
  line L480 (2.131, -59.9621) -> (2.131, -30)
  line L481 (2.131, -30) -> (47, -30)
  spline S7 degree 3 poles (19.3985, 25.9906) (19.5834, 25.9231) (19.7535, 25.8207) (20.0389, 25.5601) (20.1532, 25.4065) (20.3124, 25.0696) (20.3581, 24.8908) (20.3767, 24.5326) (20.352, 24.3568) (20.259, 24.0918) (20.2125, 23.9972) (20.099, 23.8235) (20.033, 23.7447) (19.9581, 23.6748) knots 0 0 0 0 0.059039 0.059039 0.116033 0.116033 0.170983 0.170983 0.223888 0.223888 0.255505 0.255505 0.286347 0.286347 0.286347 0.286347
  line L482 (-39, -18.088) -> (-37.5, -20.6861)
  line L483 (-37.5, -20.6861) -> (-34.5, -20.6861)
  line L484 (-34.5, -20.6861) -> (-33, -18.088)
  line L485 (-33, -18.088) -> (-34.5, -15.4899)
  line L486 (-37.5, -15.4899) -> (-39, -18.088)
  line L487 (-34.5, -15.4899) -> (-37.5, -15.4899)
  line L488 (-34.5, -14.4901) -> (-33, -11.892)
  line L489 (-33, -11.892) -> (-34.5, -9.2939)
  line L490 (-34.5, -9.2939) -> (-37.5, -9.2939)
  line L491 (-37.5, -9.2939) -> (-39, -11.892)
  line L492 (-37.5, -14.4901) -> (-34.5, -14.4901)
  line L493 (-39, -11.892) -> (-37.5, -14.4901)
  line L494 (-33, -5.696) -> (-34.5, -3.0979)
  line L495 (-34.5, -3.0979) -> (-37.5, -3.0979)
  line L496 (-37.5, -3.0979) -> (-39, -5.696)
  line L497 (-39, -5.696) -> (-37.5, -8.2941)
  line L498 (-34.5, -8.2941) -> (-33, -5.696)
  line L499 (-37.5, -8.2941) -> (-34.5, -8.2941)
  line L500 (-34.5, -2.0981) -> (-33, 0.5)
  line L501 (-33, 0.5) -> (-34.5, 3.0981)
  line L502 (-34.5, 3.0981) -> (-37.5, 3.0981)
  line L503 (-37.5, 3.0981) -> (-39, 0.5)
  line L504 (-37.5, -2.0981) -> (-34.5, -2.0981)
  line L505 (-39, 0.5) -> (-37.5, -2.0981)
  line L506 (-33, 6.696) -> (-34.5, 9.2941)
  line L507 (-34.5, 9.2941) -> (-37.5, 9.2941)
  line L508 (-37.5, 9.2941) -> (-39, 6.696)
  line L509 (-39, 6.696) -> (-37.5, 4.0979)
  line L510 (-34.5, 4.0979) -> (-33, 6.696)
  line L511 (-37.5, 4.0979) -> (-34.5, 4.0979)
  line L512 (-33, 12.892) -> (-34.5, 15.4901)
  line L513 (-34.5, 15.4901) -> (-37.5, 15.4901)
  line L514 (-37.5, 15.4901) -> (-39, 12.892)
  line L515 (-39, 12.892) -> (-37.5, 10.2939)
  line L516 (-34.5, 10.2939) -> (-33, 12.892)
  line L517 (-37.5, 10.2939) -> (-34.5, 10.2939)
  line L518 (-33, 19.088) -> (-34.5, 21.6861)
  line L519 (-34.5, 21.6861) -> (-37.5, 21.6861)
  line L520 (-37.5, 21.6861) -> (-39, 19.088)
  line L521 (-39, 19.088) -> (-37.5, 16.4899)
  line L522 (-34.5, 16.4899) -> (-33, 19.088)
  line L523 (-37.5, 16.4899) -> (-34.5, 16.4899)
  arc A6 (-38.6015, -23.0094) -> (-39.3985, -23.0094) centre (-39, -24.5) ccw
  arc A7 (-38.6015, 25.9906) -> (-39.3985, 25.9906) centre (-39, 24.5) ccw
  arc A8 (19.3985, -23.0094) -> (18.6015, -23.0094) centre (19, -24.5) ccw
  point P0 (36, -18.088)
  point P1 (36, -18.088)
  point P2 (30, -14.99)
  point P3 (24, -18.088)
  point P4 (36, -11.892)
  dimension "d79" = 11
  dimension "d80" = 3
  dimension "d81" = 11.912
  dimension "d82" = 5.1962
  dimension "d85" = 0
  dimension "d86" = 6.196
  dimension "d87" = 8.3139
  dimension "d88" = 9.3139
  dimension "d91" = -12
  dimension "d92" = 0
  dimension "d93" = 3
  dimension "d96" = -12
  dimension "d97" = 6.169
  dimension "d147" = 8
  dimension "d150" = -12
  dimension "d151" = 0
  dimension "d154" = 8
  constraint coincident P1 P0
  constraint parallel L3 L5
  constraint parallel L261 L262
  constraint coincident P2 L263.start
  constraint midpoint P3 L264
  constraint coincident P3 L265.end
  constraint equal L263 L265
  constraint coincident L266 P4
  constraint midpoint L266 P4
  constraint coincident P4 L267.start
  constraint equal L263 L267
  measures "d79" distance of L0 P1
  measures "d80" distance of L4.start P1
  measures "d81" distance of L3 P1
  measures "d82" distance of L5 L8
  measures "d87" distance of L1 L43
  measures "d88" distance of L3 L5
  measures "d93" distance of L256.start P2
  measures "d147" distance of L0 L11.end
  measures "d154" distance of L2 L482.start
extrude "Extrude5" cut sketch "Hexagon Air Holes" against normal through all contours L4 L5 L6 L7 L8 L9 | L10 L15 L266 L267 | L11 L12 L13 L266 | L14 L15 L266 L267 | L16 L17 L18 L19 L20 L21 | L22 L23 L24 L25 L26 L27 | L28 L29 L30 L31 L32 L33 | L34 L35 L36 L37 L38 L39 | L40 L41 L42 L43 L44 L45 | L46 L47 L50 L264 | L49 L51 L264 L265 | L48 L49 L264 L265 | L52 L53 L54 L55 L56 L57 | L58 L59 L60 L61 L62 L63 | L64 L65 L66 L67 L68 L69 | L70 L71 L72 L73 L74 L75 | L76 L77 L78 L79 L80 L81 | L82 L83 L84 L85 L86 L87 | L88 L89 L90 L91 L92 L93 | L94 L95 L96 L97 L98 L99 | L100 L101 L102 L103 L104 L105 | L106 L107 L108 L109 L110 L111 | L112 L113 L114 L115 L116 L117 | L118 L119 L120 L121 L122 L123 | L124 L125 L126 L127 L128 L129 | L130 L131 L132 L133 L134 L135 | L136 L137 L138 L139 L140 L141 | L142 L143 L144 L145 L146 L147 | L148 L149 L150 L151 L152 L153 | L154 L155 L156 L157 L158 L159 | L160 L161 L162 L163 L164 L165 | L166 L167 L168 L169 L170 L171 | L172 L173 L174 L175 L176 L177 | L178 L179 L180 L181 L182 L183 | L184 L185 L186 L187 L188 L189 | L190 L191 L192 L193 L194 L195 | L196 L197 L198 L199 L200 L201 | L202 L203 L204 L205 L206 L207 | L208 L209 L210 L211 L212 L213 | L214 L215 L216 L217 L218 L219 | L220 L221 L222 L223 L224 L225 | L226 L227 L228 L229 L230 L231 | L232 L233 L234 L235 L236 L237 | L238 L239 L240 L241 L242 L243 | L244 L245 L246 L247 L248 L249 | L250 L251 L252 L253 L254 L255 | L256 L260 L261 L263 L265 | L256 L257 L263 L267 | L257 L258 L259 L260 L265 L267 | L268 L269 L270 L271 L272 L273 | L274 L275 L276 L277 L278 L279 | L280 L281 L282 L283 L284 L285 | L286 L287 L288 L289 L290 L291 | L292 L293 L294 L295 L296 L297 | L298 L299 L300 L301 L302 L303 | L304 L305 L306 L307 L308 L309 | L310 L311 L312 L313 L314 L315 | L316 L317 L318 L319 L320 L321 | L322 L323 L324 L325 L326 L327 | L328 L329 L330 L331 L332 L333 | L334 L335 L336 L337 L338 L339 | L340 L341 L342 L343 L344 L345 | L346 L347 L348 L349 L350 L351 | L352 L353 L354 L355 L356 L357 | L358 L359 L360 L361 L362 L363 | L364 L365 L366 L367 L368 L369 | L370 L371 L372 L373 L374 L375 | L376 L377 L378 L379 L380 L381 | L382 L383 L384 L385 L386 L387 | L388 L389 L390 L391 L392 L393 | L394 L395 L396 L397 L398 L399 | L400 L401 L402 L403 L404 L405 | L406 L407 L408 L409 L410 L411 | L412 L413 L414 L415 L416 L417 | L418 L419 L420 L421 L422 L423 | L424 L425 L426 L427 L428 L429 | L430 L431 L432 L433 L434 L435 | L436 L437 L438 L439 L440 L441 | L442 L443 L444 L445 L446 L447 | L448 L449 L450 L451 L452 L453 | L454 L455 L456 L457 L458 L459 | L460 L461 L462 L463 L464 L465 | L466 L467 L468 L469 L470 L471 | L472 L473 L474 L475 L476 L477 | L482 L483 L484 L485 L486 L487 | L488 L489 L490 L491 L492 L493 | L494 L495 L496 L497 L498 L499 | L500 L501 L502 L503 L504 L505 | L506 L507 L508 L509 L510 L511 | L512 L513 L514 L515 L516 L517 | L518 L519 L520 L521 L522 L523